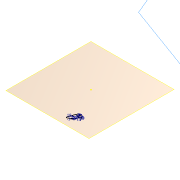
# Autodesk Inventor part: new clip
Saved by Autodesk Inventor 2016 (Build 200138000, 138)
## iProperties
Created: 2017-06-21
Part Number: new clip
Material: Generic
Document SubType Name: Modeling
Designer: Juny
Density: 1 g/cm^3
Appearance: Default
Author: Juny
Autodesk Inventor part; units mm, degrees
ref_plane "YZ Plane" through (0, 0, 0) normal (1, 0, 0) x (0, 1, 0)
ref_plane "XZ Plane" through (0, 0, 0) normal (0, 1, 0) x (-1, 0, 0)
ref_plane "XY Plane" through (0, 0, 0) normal (0, 0, 1) x (1, 0, 0)
ref_plane "Work Plane1" through (0, 0, 0) normal (0, 0, 1) x (1, 0, 0)
sketch "Sketch1" plane through (0, 0, 0) normal (0, 0, 1) x (1, 0, 0)
  circle A0 centre (55, -95.2628) radius 1.5 projected
  arc A1 (62.0359, -97.8602) -> (47.9641, -92.6654) centre (55, -95.2628) ccw
  line L0 (61.5123, -91.5426) -> (70.4408, -107.1721)
  line L1 (47.9641, -92.6654) -> (38.1093, -119.3603)
  line L2 (62.0359, -97.8602) -> (55.8021, -114.7463)
  line L3 (55.8021, -114.7463) -> (51.1115, -113.0147)
  line L4 (38.1093, -119.3603) -> (39.4539, -122.2786)
  line L5 (51.1115, -113.0147) -> (52.3818, -115.7717)
  line L6 (55.8021, -114.7463) -> (53.0451, -116.0165)
  line L7 (51.715, -116.6294) -> (39.4539, -122.2786)
  line L8 (56.3853, -91.5103) -> (53.6147, -99.0153) construction
  line L9 (57.3703, -91.874) -> (54.5997, -99.3789)
  line L10 (52.6297, -98.6516) -> (55.4003, -91.1467)
  arc A2 (57.3703, -91.874) -> (55.4003, -91.1467) centre (56.3853, -91.5103) ccw
  arc A3 (52.6297, -98.6516) -> (54.5997, -99.3789) centre (53.6147, -99.0153) ccw
  line L11 (53.0451, -116.0165) -> (52.6233, -116.2109)
  arc A4 (52.6233, -116.2109) -> (51.715, -116.6294) centre (52.1692, -116.4201) ccw
  point P0 (0, 0)
  dimension "d0" = 15
  dimension "d1" = 18
  dimension "d2" = 18
  dimension "d3" = 50
  dimension "d4" = 5
  dimension "d6" = 18
  dimension "d8" = 8
  dimension "d9" = 2.1
  dimension "d21" = 1
  dimension "d22" = 14
  constraints: 26 end point, 9 point on circle, 7 tangent, 5 perpendicular, 4 centre point, 3 parallel, 1 coincident, 1 midpoint, 1 point on line
  measures "d0" diameter of A1
  measures "d1" distance of L2.start L2.end
  measures "d2" distance of L0.start L0.end
  measures "d3" angle of L0 L2
  measures "d4" distance of L2.end L3.end
  measures "d6" distance from line of L4 L2.end
  measures "d8" distance of L8.start L8.end
  measures "d9" distance between parallel lines of L9 L10
  measures "d21" diameter of A4
  measures "d22" distance from line of L4 A4.centre
extrude "Extrusion1" add sketch "Sketch1" along normal blind 0.7
sketch "Sketch2" plane through (39.4539, -122.2786, 0) normal (-0.9082341, -0.4184624, 0) x (0, 0, 1)
  line L0 (0, 3.2132) -> (0, 0) projected
  line L1 (0, 0) -> (0.7, 0) projected
  line L2 (0.7, 3.2132) -> (0.7, 0) projected
  line L3 (0, 3.2132) -> (0.7, 3.2132) projected
  line L4 (0, 0) -> (0.7, 0) projected
  line L5 (0, 0) -> (-6.5, 0)
  line L6 (-6.5, 0) -> (-6.5, 0.7)
  line L7 (-6.5, 0.7) -> (0, 0.7)
  line L8 (0, 0.7) -> (0, 0)
  line L9 (-6.5, 0.7) -> (-5.8106, 0.5784)
  line L10 (-5.8106, 0.5784) -> (-4.7687, 6.4873)
  line L11 (-4.7687, 6.4873) -> (-5.4581, 6.6088)
  line L12 (-5.4581, 6.6088) -> (-6.5, 0.7)
  line L13 (-4.7687, 6.4873) -> (-5.2831, 6.1271)
  line L14 (-5.2831, 6.1271) -> (-7.0039, 8.5846)
  line L15 (-7.0039, 8.5846) -> (-6.4895, 8.9447)
  line L16 (-6.4895, 8.9447) -> (-4.7687, 6.4873)
  point P0 (0, 127.5676)
  dimension "d12" = 6
  dimension "d13" = 6.5
  dimension "d14" = 0.7
  dimension "d15" = 0.7
  dimension "d16" = 3
  dimension "d17" = 80
  dimension "d18" = 135
  constraints: 24 end point, 6 parallel, 3 perpendicular, 1 horizontal
  measures "d12" distance between parallel lines of L9 L11
  measures "d13" distance between parallel lines of L0 L6
  measures "d14" distance between parallel lines of L5 L7
  measures "d15" distance between parallel lines of L12 L10
  measures "d16" distance of L13.end L14.end
  measures "d17" angle of L7 L10
  measures "d18" angle of L12 L14
extrude "Extrusion2" add sketch "Sketch2" against normal blind 13.5 contours L0 L5 L6 L9 L10 L7 | L10 L9 L7 | L7 L12 L14 L13 L10 | L13 L14 L12 L11 | L11 L12 L14 L15 L16
fillet "Fillet1" radius 5 1 edges at (55.8021, -114.7463, 0.35)
fillet "Fillet2" radius 0.5 3 edges at (45.2915, -118.8182, 0) (45.2915, -118.8182, -5.7892) (42.8964, -113.6198, -5.4908)
fillet "Fillet3" radius 0.5 4 edges at (45.5845, -119.454, -6.5) (45.5845, -119.454, 0.7) (45.2915, -118.8182, -6.5) (42.8698, -113.562, -4.7687)
fillet "Fillet4" radius 2 2 edges at (48.0474, -108.669, -6.7467) (35.7862, -114.3183, -6.7467)
body "Solid1"
